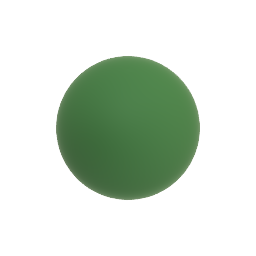
Ball (Autodesk Fusion 360 design; units mm, degrees)
Autodesk Fusion 360 part; units mm, degrees
sphere "SpherePrimitive1" add diameter 40 placed x (1, 0, 0) y (0, 1, 0) z (0, 0, 1) at (0, 0, 0) makes body 1 in component "Ball"
sketch "Sketch1" plane through (0, 0, 0) normal (0, 0, 1) x (1, 0, 0) in component "Ramp"
  line L0 (-60, 30) -> (60, 30)
  line L1 (60, 30) -> (60, -30)
  line L2 (60, -30) -> (-60, -30)
  line L3 (-60, -30) -> (-60, 30)
  line L4 (-60, 30) -> (60, -30) construction
  line L5 (60, 30) -> (-60, -30) construction
  dimension "d2" = 120
  dimension "d3" = 60
  constraint horizontal L0
  constraint perpendicular L0 L1
  constraint parallel L0 L2
  constraint parallel L1 L3
  constraint coincident L4 origin
  constraint coincident L5 origin
  measures "d2" distance of L1.end L2.end
  measures "d3" distance of L0.end L1.end
extrude "Extrude1" add sketch "Sketch1" along normal blind 50 separate body makes body 2 in component "Ramp"
sketch "Sketch2" plane through (-60, 0, 0) normal (-1, 0, 0) x (0, -1, 0) in component "Ramp"
  line L0 (-30, 0) -> (30, 0)
  line L1 (30, 0) -> (30, 50)
  line L2 (30, 50) -> (-30, 50)
  line L3 (-30, 50) -> (-30, 0)
  circle A0 centre (0, 50) radius 25
  dimension "d6" = 50
  constraint midpoint L2 A0.centre
  measures "d6" diameter of A0
extrude "Extrude2" cut sketch "Sketch2" against normal blind 140 contours L2 A0 picked at (-4.1667, 42.7831) bodies 2 in component "Ramp"
extrude "Extrude3" add 1 faces at (20, -10, 0) along direction (0, 0, -1) blind 10 on bodies 2 bodies 2 in component "Ramp"
sketch "Sketch3" plane through (60, 0, 0) normal (1, 0, 0) x (0, 1, 0) in component "Ramp"
  arc A0 (-25, 50) -> (25, 50) centre (0, 50) ccw
  line L0 (-25, 50) -> (-30, 50)
  line L1 (-30, 50) -> (-30, -10)
  line L2 (-30, -10) -> (30, -10)
  line L3 (30, -10) -> (30, 50)
  line L4 (30, 50) -> (25, 50)
  circle A1 centre (-30, 50) radius 60
  circle A2 centre (30, 50) radius 60
  constraint coincident L0.end L1.start
  constraint coincident L3.end A1
  constraint coincident L3.end L4.start
  constraint coincident L0.end A2
extrude "Extrude4" cut sketch "Sketch3" against normal blind 165 contours L1 A1 A2 | L3 A1 A2 | L2 A1 A2 picked at (-21.1858, 5.1301) picked at (21.1858, 5.1301) bodies 2 in component "Ramp"
fillet "Fillet1" radius 15 1 edges at (0, 0, -1.9615) on bodies 2 in component "Ramp"
fillet "Fillet2" radius 2.5 4 edges at (0, -30, 50) (0, -25, 50) (0, 25, 50) (0, 30, 50) on bodies 2 in component "Ramp"
move_body "MoveFace1" bodies 1 to x (1, 0, 0) y (0, 1, 0) z (0, 0, 1) at (0, 0, 46) on bodies 1 in component "Ball"
component "Ball" placed x (1, 0, 0) y (0, 1, 0) z (0, 0, 1) at (0, 0, 0)
